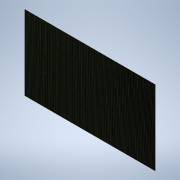
# Autodesk Inventor part: QJcell
Saved by Autodesk Inventor 2022 (Build 260153000, 153)
## iProperties
Created: 2022-02-12
Part Number: QJcell
Material: Generic
Document SubType Name: Modeling
Designer: Bowen
Density: 1 g/cm^3
Appearance: Glossy - Black
Author: Bowen
Autodesk Inventor part; units mm, degrees
ref_plane "YZ Plane" through (0, 0, 0) normal (1, 0, 0) x (0, 1, 0)
ref_plane "XZ Plane" through (0, 0, 0) normal (0, 1, 0) x (-1, 0, 0)
ref_plane "XY Plane" through (0, 0, 0) normal (0, 0, 1) x (1, 0, 0)
sketch "Sketch1" plane through (0, 0, 0) normal (0, 0, 1) x (1, 0, 0)
  line L0 (-34.55, 19.85) -> (34.55, 19.85)
  line L1 (34.55, 19.85) -> (34.55, -19.85)
  line L2 (34.55, -19.85) -> (-34.55, -19.85)
  line L3 (-34.55, -19.85) -> (-34.55, 19.85)
  point P0 (0, 0)
  point P1 (0, 0)
  point P2 (34.55, 0)
  point P3 (0, 19.85)
  dimension "d28" = 69.1
  dimension "d29" = 39.7
  constraints: 8 end point, 2 midpoint, 2 parallel, 1 coincident, 1 horizontal, 1 horizontal alignment, 1 perpendicular, 1 vertical alignment
  measures "d28" distance of L1.end L2.end
  measures "d29" distance of L0.end L1.end
extrude "Extrusion1" add sketch "Sketch1" along normal mid plane 0.11
sketch "Sketch2" plane through (0, 0, 0.055) normal (0, 0, 1) x (1, 0, 0)
  line L0 (-59.8379, 27.7762) -> (59.8379, 27.7762) construction
  line L1 (59.8379, 27.7762) -> (59.8379, -27.7762) construction
  line L2 (59.8379, -27.7762) -> (-59.8379, -27.7762) construction
  line L3 (-59.8379, -27.7762) -> (-59.8379, 27.7762) construction
  point P0 (0, 0)
  point P1 (59.8379, 0)
  point P2 (0, 27.7762)
  constraints: 2 midpoint, 1 horizontal, 1 horizontal alignment, 1 vertical alignment, 2 other
decal "Decal1"
body "Solid1"
